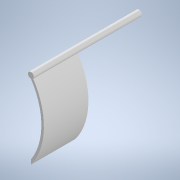
# Autodesk Inventor part: локатор
Saved by Autodesk Inventor 2021.1 (Build 251245010, 245A)
## iProperties
Created: 2023-01-21
Part Number: локатор
Material: Типовые
Document SubType Name: Modeling
Designer: zmoze
Density: 1 g/cm^3
Appearance: По умолчанию
Author: zmoze
Autodesk Inventor part; units mm, degrees
ref_plane "YZ Plane" through (0, 0, 0) normal (1, 0, 0) x (0, 1, 0)
ref_plane "XZ Plane" through (0, 0, 0) normal (0, 1, 0) x (-1, 0, 0)
ref_plane "XY Plane" through (0, 0, 0) normal (0, 0, 1) x (1, 0, 0)
sketch "Эскиз1" plane through (0, 0, 0) normal (0, 0, 1) x (1, 0, 0)
  circle A0 centre (0, 0) radius 4.6
  dimension "d0" = 9.2
  constraints: 1 centre point, 1 coincident
  measures "d0" diameter of A0
extrude "Выдавливание1" add sketch "Эскиз1" along normal blind 170
sketch "Эскиз3" plane through (0, 0, 170) normal (0, 0, 1) x (1, 0, 0)
  circle A0 centre (0, 0) radius 4.6 projected
  arc A1 (0, -114.6) -> (0, -4.6) centre (-83.8186, -59.6) ccw
  arc A2 (0, -121.5921) -> (3.6237, -2.8336) centre (-83.8186, -59.6) ccw
  line L0 (0, 0) -> (0, -4.6) construction
  line L1 (0, -114.6) -> (0, -121.5921)
  dimension "d3" = 4
  dimension "d4" = 110
  constraints: 6 point on circle, 4 end point, 2 centre point, 2 vertical, 1 collinear
  measures "d3" radial gap between concentric circles of A1 A2
  measures "d4" distance of L0.end L1.start
extrude "Выдавливание2" add sketch "Эскиз3" against normal blind 70 contours A0 A2 L1 A1
sketch "Эскиз5" plane through (0, 0, 0) normal (0, 0, -1) x (-1, 0, 0)
  line L0 (-1.5, 1.3229) -> (-1.5, -1.3229) projected
  arc A0 (1.5, 1.3229) -> (-1.5, 1.3229) centre (0, 0) ccw projected
  line L1 (1.5, -1.3229) -> (1.5, 1.3229) projected
  arc A1 (-1.5, -1.3229) -> (1.5, -1.3229) centre (0, 0) ccw projected
  point P0 (0, 0)
extrude "Выдавливание4" cut sketch "Эскиз5" against normal blind 8.4
sketch "Эскиз6" plane through (0, 0, 0) normal (0, 0, -1) x (-1, 0, 0)
  circle A0 centre (0, 0) radius 2.5 projected
  point P0 (0, 0)
extrude "Выдавливание5" cut sketch "Эскиз6" against normal blind 2.4
